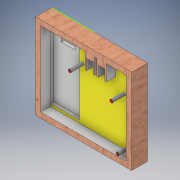
# Autodesk Inventor part: case_bottom
Saved by Autodesk Inventor 2017 (Build 210142000, 142)
## iProperties
Created: 2016-11-05
Part Number: case_bottom
Material: Generic
Document SubType Name: Modeling
Designer: radrajith
Density: 1 g/cm^3
Appearance: Default
Author: radrajith
Autodesk Inventor part; units mm, degrees
ref_plane "YZ Plane" through (0, 0, 0) normal (1, 0, 0) x (0, 1, 0)
ref_plane "XZ Plane" through (0, 0, 0) normal (0, 1, 0) x (-1, 0, 0)
ref_plane "XY Plane" through (0, 0, 0) normal (0, 0, 1) x (1, 0, 0)
sketch "Sketch1" plane through (0, 0, 0) normal (0, 0, 1) x (1, 0, 0)
  line L0 (-5, -5) -> (85, -5)
  line L1 (85, -5) -> (85, 75)
  line L2 (85, 75) -> (-5, 75)
  line L3 (-5, 75) -> (-5, -5)
  point P0 (0, 0)
  dimension "d0" = 90
  dimension "d1" = 80
  constraints: 8 end point, 2 parallel, 1 horizontal, 1 perpendicular
  measures "d0" distance of L2.end L1.end
  measures "d1" distance of L1.end L0.end
extrude "Extrusion1" add sketch "Sketch1" along normal blind 15
sketch "Sketch3" plane through (0, 0, 15) normal (0, 0, 1) x (1, 0, 0)
  line L0 (-0.1584, 0.1549) -> (79.8416, 0.1549)
  line L1 (79.8416, 0.1549) -> (79.8416, 70.1549)
  line L2 (79.8416, 70.1549) -> (-0.1584, 70.1549)
  line L3 (-0.1584, 70.1549) -> (-0.1584, 0.1549)
  point P0 (0, 0)
  dimension "d4" = 80
  dimension "d5" = 70
  constraints: 8 end point, 2 parallel, 1 horizontal, 1 perpendicular
  measures "d4" distance of L2.end L1.end
  measures "d5" distance of L1.end L0.end
extrude "Extrusion2" cut sketch "Sketch3" against normal blind 9
sketch "Sketch4" plane through (0, 0, 6) normal (0, 0, 1) x (1, 0, 0)
  circle A0 centre (75, 5) radius 1.55
  circle A1 centre (30, 50) radius 1.55
  circle A2 centre (68.99, 45) radius 1.55
  point P0 (0, 0)
  dimension "d8" = 3.1
  dimension "d9" = 3.1
  dimension "d10" = 3.1
  constraints: 3 centre point
  measures "d8" diameter of A0
  measures "d9" diameter of A1
  measures "d10" diameter of A2
extrude "Extrusion3" add sketch "Sketch4" along normal blind 12
sketch "Sketch9" plane through (0, 0, 6) normal (0, 0, 1) x (1, 0, 0)
  line L0 (0.0607, 67.5504) -> (27.0607, 67.5504)
  line L1 (27.0607, 67.5504) -> (27.0607, 2.5504)
  line L2 (27.0607, 2.5504) -> (0.0607, 2.5504)
  line L3 (0.0607, 2.5504) -> (0.0607, 67.5504)
  point P0 (0, 0)
  dimension "d13" = 27
  dimension "d14" = 65
  constraints: 8 end point, 2 parallel, 1 horizontal, 1 perpendicular
  measures "d13" distance of L1.end L2.end
  measures "d14" distance of L0.end L1.end
extrude "Extrusion4" cut sketch "Sketch9" against normal blind 3
sketch "Sketch10" plane through (0, 0, 3) normal (0, 0, 1) x (1, 0, 0)
  line L0 (7, 62.6613) -> (20, 62.6613)
  line L1 (20, 62.6613) -> (20, 54.4354)
  line L2 (20, 54.4354) -> (7, 54.4354)
  line L3 (7, 54.4354) -> (7, 62.6613)
  point P0 (0, 0)
  constraints: 8 end point, 2 parallel, 1 horizontal, 1 perpendicular
extrude "Extrusion5" cut sketch "Sketch10" against normal blind 3
sketch "Sketch12" plane through (-0.1584, 70.1549, 15) normal (0, -1, 0) x (1, 0, 0)
  line L0 (0, 0) -> (80, 0) projected
  line L1 (61.5, 0) -> (52.5, 0)
  line L2 (52.5, 0) -> (52.5, -9)
  line L3 (52.5, -9) -> (61.5, -9)
  line L4 (61.5, -9) -> (61.5, 0)
  line L5 (50.5, 0) -> (41.5, 0)
  line L6 (41.5, 0) -> (41.5, -9)
  line L7 (41.5, -9) -> (50.5, -9)
  line L8 (50.5, -9) -> (50.5, 0)
  point P0 (0.1584, -15)
  constraints: 16 end point, 4 parallel, 2 horizontal, 2 perpendicular
extrude "Extrusion7" add sketch "Sketch12" along normal blind 15
sketch "Sketch13" plane through (-0.1584, 55.1549, 15) normal (0, -1, 0) x (1, 0, 0)
  line L0 (61.5, 0) -> (52.5, 0) projected
  line L1 (60, 0) -> (54, 0)
  line L2 (54, 0) -> (54, -8)
  line L3 (54, -8) -> (60, -8)
  line L4 (60, -8) -> (60, 0)
  line L5 (50.5, 0) -> (41.5, 0) projected
  line L6 (49, 0) -> (43, 0)
  line L7 (43, 0) -> (43, -8)
  line L8 (43, -8) -> (49, -8)
  line L9 (49, -8) -> (49, 0)
  point P0 (0.1584, -15)
  constraints: 16 end point, 4 parallel, 2 horizontal, 2 perpendicular, 1 point on line
extrude "Extrusion8" cut sketch "Sketch13" against normal blind 10
sketch "Sketch14" plane through (0, 0, 0) normal (0, 0, -1) x (-1, 0, 0)
  line L0 (-85, -5) -> (5, -5) projected
  line L1 (-35, -5) -> (4.5, -5)
  line L2 (4.5, -5) -> (4.5, 75)
  line L3 (4.5, 75) -> (-35, 75)
  line L4 (-35, 75) -> (-35, -5)
  point P0 (0, 0)
  constraints: 8 end point, 2 parallel, 1 horizontal, 1 perpendicular, 1 point on line
thread "Thread1" size "M3.5x0.6" class "6g" standard "ANSI Metric M Profile" full length
thread "Thread2" size "M3.5x0.6" class "6g" standard "ANSI Metric M Profile" full length
thread "Thread3" size "M3.5x0.6" class "6g" standard "ANSI Metric M Profile" full length
body "Solid1"
